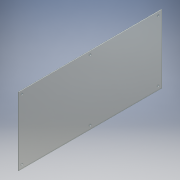
# Autodesk Inventor part: long covering
Saved by Autodesk Inventor 2016 (Build 200138000, 138)
## iProperties
Created: 2016-08-02
Part Number: long covering
Material: Glass
Document SubType Name: Modeling
Designer: Jonathan
Density: 2.18 g/cm^3
Appearance: Clear
Author: Jonathan
Autodesk Inventor part; units mm, degrees
ref_plane "YZ Plane" through (0, 0, 0) normal (1, 0, 0) x (0, 1, 0)
ref_plane "XZ Plane" through (0, 0, 0) normal (0, 1, 0) x (-1, 0, 0)
ref_plane "XY Plane" through (0, 0, 0) normal (0, 0, 1) x (1, 0, 0)
sketch "Sketch1" plane through (0, 0, 0) normal (1, 0, 0) x (0, 1, 0)
  line L0 (200, 95) -> (-200, 95)
  line L1 (-200, 95) -> (-200, -95)
  line L2 (-200, -95) -> (200, -95)
  line L3 (200, -95) -> (200, 95)
  line L4 (200, 95) -> (-200, -95) construction
  line L5 (-200, 95) -> (200, -95) construction
  point P0 (0, 0)
  dimension "d0" = 400
  dimension "d1" = 190
  constraints: 12 end point, 2 midpoint, 2 parallel, 1 horizontal, 1 perpendicular
  measures "d0" distance of L1.end L2.end
  measures "d1" distance of L2.end L0.start
extrude "Extrusion1" add sketch "Sketch1" along normal blind 1.5875
sketch "Sketch2" plane through (1.5875, 0, 0) normal (1, 0, 0) x (0, 0, -1)
  circle A0 centre (-85, 190) radius 5
  circle A1 centre (85, 190) radius 5
  circle A2 centre (85, -190) radius 5
  circle A3 centre (-85, -190) radius 5
  line L0 (95, 200) -> (-95, 200) projected
  line L1 (-95, 200) -> (-95, -200) projected
  line L2 (-95, -200) -> (95, -200) projected
  line L3 (95, -200) -> (95, 200) projected
  point P0 (0, 0)
  point P1 (-85, 0)
  point P2 (85, 0)
  dimension "d4" = 10
  dimension "d5" = 10
  dimension "d6" = 10
  dimension "d7" = 10
  dimension "d8" = 10
  constraints: 4 centre point, 4 horizontal alignment, 4 vertical alignment, 3 equal radius
  measures "d4" distance from line of L0 A0.centre
  measures "d5" distance from line of L1 A0.centre
  measures "d6" distance from line of L2 A3.centre
  measures "d7" distance from line of L3 A1.centre
  measures "d8" diameter of A0
hole "Hole1" at (1.5875, 190, 85) at (1.5875, 190, -85) at (1.5875, -190, -85) at (1.5875, -190, 85) at (1.5875, 0, 85) at (1.5875, 0, -85) direction (-1, 0, 0) diameter 5.5 end through all clearance for "Flat Head Machine Screw" size "M5" standard "Ansi Metric M Profile"
body "Solid1"
